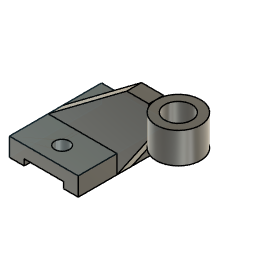
ORTHOGRAPHIC PROJECTIONS_MODEL_3 (Autodesk Fusion 360 design; units mm, degrees)
Autodesk Fusion 360 part; units mm, degrees
sketch "Sketch1" plane through (0, 0, 0) normal (0, 1, 0) x (1, 0, 0)
  line L0 (-28, 0) -> (-28, -7.5)
  line L1 (-28, -7.5) -> (28, -7.5)
  line L2 (28, -7.5) -> (28, 7.5)
  line L3 (-28, 0) -> (-28, 7.5)
  line L4 (-28, 7.5) -> (-16, 7.5)
  line L5 (-16, 7.5) -> (-16, 2.5)
  line L6 (-16, 2.5) -> (16, 2.5)
  line L7 (16, 2.5) -> (16, 7.5)
  line L8 (16, 7.5) -> (28, 7.5)
  dimension "d3" = 7.5
  dimension "d4" = 56
  dimension "d5" = 15
  dimension "d6" = 7.5
  dimension "d7" = 12
  dimension "d8" = 5
  dimension "d9" = 32
  dimension "d10" = 5
  constraint perpendicular L0 L1
  constraint perpendicular L3 L4
  constraint perpendicular L4 L5
  constraint perpendicular L5 L6
  constraint perpendicular L6 L7
  measures "d3" distance of L0.start L0.end
  measures "d4" distance of L0.end L1.end
  measures "d5" distance of L1.end L2.end
  measures "d6" distance of L0.start L3.end
  measures "d7" distance of L3.end L4.end
  measures "d8" distance of L4.end L5.end
  measures "d9" distance of L5.end L6.end
  measures "d10" distance of L6.end L7.end
sketch "Sketch2" plane through (28, 0, 0) normal (1, 0, 0) x (0, 1, 0)
sketch "Sketch3" plane through (-28, 0, 0) normal (-1, 0, 0) x (0, -1, 0)
sketch "Sketch4" plane through (0, 0, 0) normal (0, 1, 0) x (1, 0, 0)
  line L0 (0, 0) -> (0, -7.5)
  line L1 (0, -7.5) -> (-28, -7.5)
  line L2 (-28, -7.5) -> (-28, 7.5)
  line L3 (-28, 7.5) -> (-16, 7.5)
  line L4 (-16, 7.5) -> (-16, 2.5)
  line L5 (-16, 2.5) -> (16, 2.5)
  line L6 (16, 2.5) -> (16, 7.5)
  line L7 (16, 7.5) -> (28, 7.5)
  line L8 (28, 7.5) -> (28, -7.5)
  line L9 (28, -7.5) -> (0, -7.5)
  dimension "d19" = 7.5
  dimension "d20" = 28
  dimension "d21" = 15
  dimension "d22" = 12
  dimension "d23" = 5
  dimension "d24" = 32
  dimension "d25" = 5
  dimension "d26" = 12
  constraint coincident L0.start origin
  constraint vertical L0
  constraint perpendicular L0 L1
  constraint perpendicular L1 L2
  constraint perpendicular L2 L3
  constraint perpendicular L3 L4
  constraint perpendicular L4 L5
  constraint perpendicular L5 L6
  constraint perpendicular L6 L7
  constraint perpendicular L1 L8
  constraint perpendicular L0 L9
  measures "d19" distance of L0.start L0.end
  measures "d20" distance of L0.end L1.end
  measures "d21" distance of L1.end L2.end
  measures "d22" distance of L2.end L3.end
  measures "d23" distance of L3.end L4.end
  measures "d24" distance of L4.end L5.end
  measures "d25" distance of L5.end L6.end
  measures "d26" distance of L6.end L7.end
extrude "Extrude2" add sketch "Sketch4" along normal mid plane 75 makes body 1
sketch "Sketch5" plane through (0, -37.5, 0) normal (0, -1, 0) x (1, 0, 0)
  line L0 (28, -7.5) -> (28, 7.5)
  line L1 (28, 7.5) -> (-28, 7.5)
  line L2 (-28, 7.5) -> (-28, -7.5)
  line L3 (-28, -7.5) -> (-16, -7.5)
  line L4 (-16, -7.5) -> (-16, -2.5)
  line L5 (-16, -2.5) -> (16, -2.5)
  line L6 (16, -2.5) -> (16, -7.5)
  line L7 (16, -7.5) -> (28, -7.5)
  line L8 (-28, -7.5) -> (-28, 7.5)
  line L9 (36, 55.5) -> (54, 55.5)
  line L10 (54, 55.5) -> (36, 55.5)
  line L11 (-28, 7.5) -> (36, 55.5)
  line L12 (36, 55.5) -> (54, 55.5)
  line L13 (54, 55.5) -> (54, 30.5)
  line L14 (54, 30.5) -> (28, -7.5)
  dimension "d32" = 18
  dimension "d33" = 25
  constraint coincident L2.end L3.start
  constraint perpendicular L3 L8
  constraint perpendicular L8 L9
  constraint parallel L9 L10
  constraint coincident L1.end L2.start
  constraint parallel L10 L12
  constraint perpendicular L12 L13
  constraint coincident L0.start L7.end
  measures "d32" distance of L9.start L9.end
  measures "d33" distance of L9.end L13.end
extrude "Extrude3" add sketch "Sketch5" along normal blind 12 separate body contours L0 L1 L9 L10 L11 L12 L13 L14 makes body 2
sketch "Sketch6" plane through (-28, 0, 0) normal (-1, 0, 0) x (0, -1, 0)
  line L0 (37.5, 7.5) -> (-37.5, 7.5)
  line L1 (-37.5, 7.5) -> (-37.5, -7.5)
  line L2 (-37.5, -7.5) -> (37.5, -7.5)
  line L3 (37.5, -7.5) -> (37.5, 7.5)
sketch "Sketch7" plane through (0, 0, 7.5) normal (0, 0, 1) x (-1, 0, 0)
  line L0 (-28, 37.5) -> (-28, -37.5)
  line L1 (-28, -37.5) -> (28, -37.5)
  line L2 (28, -37.5) -> (28, 37.5)
  line L3 (28, 37.5) -> (-28, 37.5)
move_body "Move1" bodies 2 to x (1, 0, 0) y (0, 1, 0) z (0, 0, 1) at (0, 43.5, 0)
sketch "Sketch8" plane through (0, 0, 55.5) normal (0, 0, 1) x (-1, 0, 0)
  line L0 (-54, -6) -> (-36, -6)
  line L1 (-36, -6) -> (-36, 6)
  line L2 (-36, 6) -> (-54, 6)
  line L3 (-54, 6) -> (-54, -6)
  line L4 (-54, 0) -> (-72, 0)
  circle A0 centre (-72, 0) radius 18
  circle A1 centre (-72, 0) radius 11
  dimension "d36" = 18
  dimension "d37" = 22
  constraint midpoint L3 L4.start
  constraint perpendicular L3 L4
  constraint coincident L4.end A0.centre
  constraint coincident L4.start A0
  measures "d36" distance of L4.start L4.end
  measures "d37" diameter of A1
extrude "Extrude4" add sketch "Sketch8" against normal blind 25 separate body contours A0 makes body 3
sketch "Sketch9" plane through (0, 0, 7.5) normal (0, 0, 1) x (-1, 0, 0)
  circle A0 centre (0.1468, 22.5165) radius 6
  circle A1 centre (-0.0427, -22.1376) radius 6
  dimension "d42" = 12
  dimension "d45" = 12
  measures "d42" diameter of A0
  measures "d45" diameter of A1
extrude "Extrude5" cut sketch "Sketch9" against normal blind 10 bodies 1
combine "Combine1" operation add target body 2 tool bodies 3
